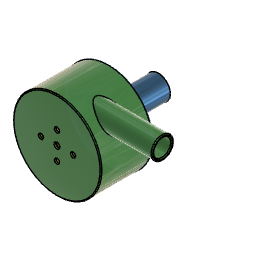
BLDC-WP main (Autodesk Fusion 360 design; units mm, degrees)
Autodesk Fusion 360 part; units mm, degrees
note: some values were not read from the file. Chosen so that the rebuilt part matches the saved one: which face or edge a step refers to; which pieces of a blend or face edit are solid. Set by a fixed rule: which sketch regions a step uses.
sketch "Sketch1" plane through (0, 0, 0) normal (0, 1, 0) x (1, 0, 0) in component "P1"
  circle A0 centre (0, 0) radius 26
  dimension "d1" = 52
  constraint coincident A0.centre origin
  measures "d1" diameter of A0
extrude "Extrude1" add sketch "Sketch1" along normal blind 2 makes body 1 in component "P1"
sketch "Sketch2" plane through (0, 0, 0) normal (0, -1, 0) x (1, 0, 0) in component "P1"
  circle A0 centre (0, 0) radius 26
  line L0 (0, 0) -> (9.5, 0) construction
  line L1 (0, 0) -> (0, 8) construction
  circle A1 centre (0, 8) radius 1.5
  circle A2 centre (9.5, 0) radius 1.5
  circle A3 centre (0, -8) radius 1.5
  circle A4 centre (-9.5, 0) radius 1.5
  dimension "d4" = 9.5
  dimension "d5" = 8
  dimension "d6" = 3
  dimension "d7" = 3
  constraint coincident A0.centre L0.start
  constraint horizontal L0
  constraint perpendicular L0 L1
  constraint coincident L1.end A1.centre
  constraint coincident L0.end A2.centre
  constraint symmetric L0 A1 A3
  constraint symmetric L1 A2 A4
  measures "d4" distance of A0.centre L0.end
  measures "d5" distance of A0.centre L1.end
  measures "d6" diameter of A1
  measures "d7" diameter of A2
extrude "Extrude2" cut sketch "Sketch2" against normal blind 15 contours A1 | A2 | A3 | A4 bodies 1 in component "P1"
chamfer "Chamfer1" distance 0.01 angle 45 4 edges at (-10.8985, 0, 0.5424) (-1.3985, 0, -7.4576) (8.1015, 0, 0.5424) (-1.3985, 0, 8.5424) on bodies 1 in component "P1"
sketch "Sketch3" plane through (0, 0, 0) normal (0, 1, 0) x (1, 0, 0) in component "P1"
  circle A0 centre (0, 0) radius 26
  circle A1 centre (0, 0) radius 24
  dimension "d11" = 52
  dimension "d12" = 48
  constraint coincident A0.centre A1.centre
  measures "d11" diameter of A0
  measures "d12" diameter of A1
extrude "Extrude3" add sketch "Sketch3" along normal blind 26 bodies 1 in component "P1"
ref_plane "WorkPlane1" through (50, 0, 0) normal (1, 0, 0) x (0, 1, 0) in component "P1"
sketch "Sketch4" plane through (50, 0, 0) normal (1, 0, 0) x (0, 1, 0) in component "P1"
  circle A0 centre (12.6606, 17.4604) radius 6.5
  circle A1 centre (12.6606, 17.4604) radius 5.1
  dimension "d16" = 13
  dimension "d17" = 10.2
  constraint concentric A0 A1
  measures "d16" diameter of A0
  measures "d17" diameter of A1
extrude "Extrude4" add sketch "Sketch4" against normal blind 50 bodies 1 in component "P1"
sketch "Sketch5" plane through (0, 26, 0) normal (0, 1, 0) x (-1, 0, 0) in component "P1"
  circle A0 centre (0, 0) radius 24
  circle A1 centre (0, 0) radius 26
  circle A2 centre (0, 0) radius 24
  dimension "d20" = 48
  constraint concentric A0 A2
  measures "d20" diameter of A2
extrude "Extrude5" cut sketch "Sketch5" against normal blind 25 contours A0 A2 bodies 1 in component "P1"
sketch "Sketch6" plane through (50, 0, 0) normal (1, 0, 0) x (0, 1, 0) in component "P1"
  circle A0 centre (12.6606, 17.4604) radius 5.1
  circle A1 centre (12.6606, 17.4604) radius 6.5
  circle A2 centre (12.6606, 17.4604) radius 5.1
  dimension "d23" = 10.2
  constraint concentric A0 A2
  measures "d23" diameter of A2
extrude "Extrude6" cut sketch "Sketch6" against normal blind 50 contours A0 A2 bodies 1 in component "P1"
sketch "Sketch7" plane through (0, 0, 0) normal (0, -1, 0) x (1, 0, 0) in component "P1"
  circle A0 centre (0, 0) radius 26
  circle A1 centre (9.5, 0) radius 1.51
  circle A2 centre (-9.5, 0) radius 1.51
  circle A3 centre (0, -8) radius 1.51
  circle A4 centre (0, 8) radius 1.51
  circle A5 centre (0, 0) radius 1.75
  dimension "d26" = 3.5
  constraint coincident A0.centre A5.centre
  measures "d26" diameter of A5
extrude "Extrude7" cut sketch "Sketch7" against normal blind 5 contours A5 bodies 1 in component "P1"
sketch "Sketch8" plane through (0, 1, 0) normal (0, 1, 0) x (-1, 0, 0) in component "P1"
  circle A0 centre (0, 0) radius 1.75
  circle A1 centre (0, 0) radius 24
  circle A2 centre (0, 8) radius 1.5
  circle A3 centre (-9.5, 0) radius 1.5
  circle A4 centre (0, -8) radius 1.5
  circle A5 centre (9.5, 0) radius 1.5
ref_plane "WorkPlane2" through (0, 3, 0) normal (0, 1, 0) x (-1, 0, 0) in component "P1"
sketch "Sketch9" plane through (0, 3, 0) normal (0, 1, 0) x (1, 0, 0) in component "P1"
  circle A0 centre (0, 0) radius 22
  dimension "d30" = 44
  constraint coincident A0.centre origin
  measures "d30" diameter of A0
extrude "Extrude8" add sketch "Sketch9" along normal blind 2 separate body makes body 2 in component "P1"
sketch "Sketch10" plane through (0, 5, 0) normal (0, 1, 0) x (-1, 0, 0) in component "P1"
  circle A0 centre (0, 0) radius 22
  line L0 (0, 0) -> (0, 22) construction
  line L1 (-1, 0) -> (-1, 20) construction
  line L2 (1, 0) -> (1, 20) construction
  circle A1 centre (0, 0) radius 6.5
  spline S0 degree 5 poles (1, 6.4226) (1.0143, 6.8807) (1.0755, 7.7684) (1.2653, 9.0147) (1.7159, 10.5048) (2.613, 12.0748) (3.8429, 13.346) (5.3916, 14.3161) (7.2214, 14.993) (9.2669, 15.3975) (11.4483, 15.5573) (13.6811, 15.503) (15.8864, 15.2645) (18.0008, 14.8683) (19.9864, 14.3345) (21.8243, 13.6777) (23.1714, 13.0611) (24.1124, 12.5495) (24.7092, 12.1868) (25, 12) knots 0 0 0 0 0 0 0.066667 0.133333 0.2 0.266667 0.333333 0.4 0.466667 0.533333 0.6 0.666667 0.733333 0.8 0.866667 0.933333 1 1 1 1 1 1
  spline S1 degree 5 poles (-1, 6.4226) (-1.0337, 6.7876) (-1.0748, 7.5036) (-1.0577, 8.5362) (-0.8767, 9.8295) (-0.3849, 11.3045) (0.3716, 12.634) (1.3857, 13.8129) (2.6402, 14.8352) (4.1048, 15.6945) (5.7297, 16.3845) (7.4511, 16.9003) (9.1977, 17.239) (10.8973, 17.4014) (12.4828, 17.3933) (13.8987, 17.2274) (15.1081, 16.925) (16.0982, 16.5177) (16.872, 16.0414) (17.4417, 15.53) (17.8215, 15.0111) (17.9809, 14.6012) (18.0212, 14.2987) (18.0129, 14.0992) (18, 14) knots 0 0 0 0 0 0 0.05 0.1 0.15 0.2 0.25 0.3 0.35 0.4 0.45 0.5 0.55 0.6 0.65 0.7 0.75 0.8 0.85 0.9 0.95 1 1 1 1 1 1
  circle A2 centre (0, 0) radius 22
  point P0 (5, 14)
  point P1 (15.8835, 15.2222)
  point P2 (3, 15)
  point P3 (13.6926, 17.2195)
  point P4 (17.4653, 15.4488)
  dimension "d37" = 1
  dimension "d38" = 1
  dimension "d39" = 13
  constraint coincident A0.centre L0.start
  constraint coincident A0 L0.end
  constraint vertical L0
  constraint vertical L1
  constraint parallel L0 L2
  constraint concentric A0 A1
  constraint coincident A1 S0.start
  constraint coincident L2 S0.start
  constraint coincident A0 P1
  constraint coincident A1 S1.start
  constraint coincident L1 S1.start
  constraint coincident A0 P3
  constraint concentric A1 A2
  measures "d37" distance of L0 L1
  measures "d38" distance of L0 L2
  measures "d39" diameter of A1
extrude "Extrude9" add sketch "Sketch10" along normal blind 10 contours A1 bodies 2 in component "P1"
extrude "Extrude10" add sketch "Sketch10" along normal blind 21 contours A0 A1 S0 S1 A2 picked at (12.0381, 16.1056) bodies 2 in component "P1"
pattern_circular "C-Pattern1" count 4 over 360 about axis through (0, 5, 0) along (0, -1, 0) of "Extrude10" in component "P1"
sketch "Sketch11" plane through (0, 3, 0) normal (0, -1, 0) x (1, 0, 0) in component "P1"
  circle A0 centre (0, 0) radius 22
  circle A1 centre (0, 0) radius 4
  dimension "d46" = 8
  constraint coincident A0.centre A1.centre
  measures "d46" diameter of A1
extrude "Extrude11" cut sketch "Sketch11" against normal blind 7 draft -10 contours A1 bodies 2 in component "P1"
sketch "Sketch12" plane through (0, 0, 0) normal (0, 1, 0) x (1, 0, 0) in component "P1"
  circle A0 centre (0, 0) radius 2.7657
  circle A1 centre (0, 0) radius 2.65
  dimension "d49" = 5.5314
  dimension "d50" = 5.3
  constraint concentric A0 A1
  measures "d49" diameter of A0
  measures "d50" diameter of A1
extrude "Extrude12" cut sketch "Sketch12" along normal blind 33 contours A1 bodies 2 in component "P1"
ref_plane "WorkPlane3" through (0, 28, 0) normal (0, 1, 0) x (0, 0, 1) in component "P1"
sketch "Sketch13" plane through (0, 28, 0) normal (0, 1, 0) x (1, 0, 0) in component "P1"
  circle A0 centre (0, 0) radius 25
  dimension "d54" = 50
  constraint coincident A0.centre origin
  measures "d54" diameter of A0
extrude "Extrude13" add sketch "Sketch13" along normal blind 2 separate body makes body 3 in component "P1"
sketch "Sketch14" plane through (0, 26, 0) normal (0, 1, 0) x (-1, 0, 0) in component "P1"
  circle A0 centre (0, 0) radius 24
  circle A1 centre (0, 0) radius 26
  circle A2 centre (0, 0) radius 24
  circle A3 centre (0, 0) radius 26
  constraint coincident A0.centre A1.centre
extrude "Extrude14" add sketch "Sketch14" along normal blind 1.9 bodies 1 in component "P1"
sketch "Sketch15" plane through (0, 27.9, 0) normal (0, 1, 0) x (-1, 0, 0) in component "P1"
  circle A0 centre (0, 0) radius 24
  circle A1 centre (0, 0) radius 26
  circle A2 centre (0, 0) radius 26
  circle A3 centre (0, 0) radius 25.05
  dimension "d59" = 50.1
  constraint coincident A0.centre A1.centre
  measures "d59" diameter of A3
extrude "Extrude15" add sketch "Sketch15" along normal blind 3 contours A1 A2 bodies 1 in component "P1"
sketch "Sketch16" plane through (0, 30.9, 0) normal (0, 1, 0) x (-1, 0, 0) in component "P1"
  circle A0 centre (0, 0) radius 25.05
  circle A1 centre (0, 0) radius 26
sketch "Sketch17" plane through (0, 30.9, 0) normal (0, 1, 0) x (-1, 0, 0) in component "P1"
  circle A0 centre (0, 0) radius 25.05
  circle A1 centre (0, 0) radius 23.5
  dimension "d62" = 50.1
  dimension "d63" = 47
  constraint coincident A0.centre A1.centre
  constraint concentric A0 A1
  measures "d62" diameter of A0
  measures "d63" diameter of A1
extrude "Extrude16" add sketch "Sketch17" against normal blind 1 bodies 1 in component "P1"
fillet "Fillet1" radius 0.5 1 edges at (21.9097, 30.9, 8.498) on bodies 1 in component "P1"
fillet "Fillet2" radius 0.5 1 edges at (21.9097, 29.9, -8.498) on bodies 1 in component "P1"
fillet "Fillet3" radius 0.5 1 edges at (24.2405, 30.9, -9.402) on bodies 1 in component "P1"
fillet "Fillet4" radius 0.5 1 edges at (-24.2405, 0, 9.402) on bodies 1 in component "P1"
fillet "Fillet5" radius 0.5 1 edges at (50, 6.6004, 15.1099) on bodies 1 in component "P1"
fillet "Fillet6" radius 0.5 1 edges at (50, 7.9057, 19.3047) on bodies 1 in component "P1"
sketch "Sketch18" plane through (0, 30.9, 0) normal (0, 1, 0) x (-1, 0, 0) in component "P1"
  circle A0 centre (0, 0) radius 7.5
  circle A1 centre (0, 0) radius 9
  dimension "d78" = 15
  dimension "d79" = 18
  constraint coincident A0.centre A1.centre
  measures "d78" diameter of A0
  measures "d79" diameter of A1
extrude "Extrude17" cut sketch "Sketch18" against normal blind 3.1 contours A0 bodies 3 in component "P1"
sketch "Sketch19" plane through (0, 0, 0) normal (0, 0, 1) x (1, 0, 0) in component "P1"
  line L0 (0, 30) -> (0, 40) construction
  line L1 (0, 40) -> (-5, 40)
  line L2 (-5, 40) -> (-7.4652, 29.6744)
  line L3 (-9.5717, 29.4637) -> (-7.0562, 40)
  line L4 (-7.0562, 40) -> (-5, 40)
  line L5 (-9.5717, 29.4637) -> (-7.4652, 29.6744)
  line L6 (-7.4652, 29.6744) -> (-9.4105, 30.1388)
  dimension "d82" = 10
  dimension "d83" = 5
  dimension "d84" = 2
  dimension "d85" = 2
  constraint vertical L0
  constraint perpendicular L0 L1
  constraint parallel L2 L3
  constraint parallel L1 L4
  constraint perpendicular L3 L6
  measures "d82" distance of L0.start L0.end
  measures "d83" distance of L0.end L1.end
  measures "d84" distance of L2 L3
  measures "d85" distance of L2.end L6.end
revolve "Revolve1" add sketch "Sketch19" angle 360 about axis through (0, 30, 0) along (0, 1, 0) contours L2 L3 L4 L6 bodies 3 in component "P1"
sketch "Sketch20" plane through (0, 40, 0) normal (0, 1, 0) x (-1, 0, 0) in component "P1"
  circle A0 centre (0, 0) radius 7.0562
  circle A1 centre (0, 0) radius 5
  circle A2 centre (0, 0) radius 7.0562
  circle A3 centre (0, 0) radius 5
  constraint concentric A0 A2
  constraint concentric A0 A3
extrude "Extrude18" add sketch "Sketch20" along normal blind 20 bodies 3 in component "P1"
sketch "Sketch1 (2)" plane through (0, 0, 0) normal (0, 1, 0) x (1, 0, 0)
component "P1" placed x (1, 0, 0) y (0, 1, 0) z (0, 0, 1) at (0, 0, 0)
